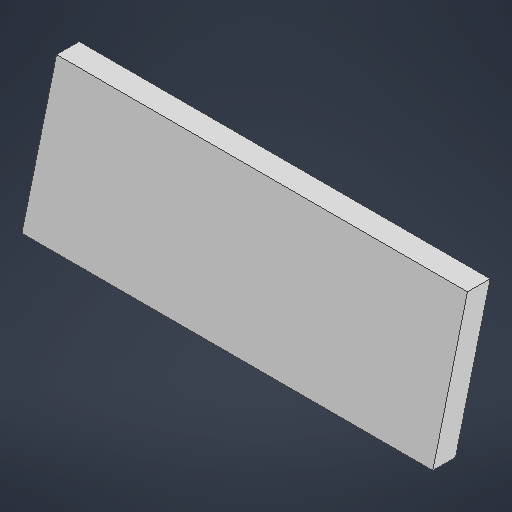
# Autodesk Inventor part: для ведра
Saved by Autodesk Inventor 2025 (Build 290162000, 162)
## iProperties
Created: 2025-03-17
Part Number: для ведра
Material: Типовые
Document SubType Name: Modeling
Designer: Phantom
Density: 1 g/cm^3
Appearance: По умолчанию
Author: Phantom
Autodesk Inventor part; units mm, degrees
ref_plane "YZ Plane" through (0, 0, 0) normal (1, 0, 0) x (0, 1, 0)
ref_plane "XZ Plane" through (0, 0, 0) normal (0, 1, 0) x (-1, 0, 0)
ref_plane "XY Plane" through (0, 0, 0) normal (0, 0, 1) x (1, 0, 0)
sketch "Эскиз1" plane through (0, 0, 0) normal (0, 0, 1) x (1, 0, 0)
  line L0 (0, 0) -> (58, 0)
  line L1 (58, 0) -> (58, 22)
  line L2 (58, 22) -> (0, 22)
  line L3 (0, 22) -> (0, 0)
  dimension "d8" = 58
  constraints: 8 end point, 2 parallel, 1 horizontal, 1 perpendicular
  measures "d8" distance of L0.start L0.end
extrude "Выдавливание1" add sketch "Эскиз1" along normal blind 3.2
sketch "Эскиз2" plane through (0, 0, 0) normal (-1, 0, 0) x (0, 0, 1)
  line L0 (-8.3013, 45.5697) -> (3.4651, -1.0505)
  line L1 (45.6651, 0) -> (-10.7349, 0)
  line L2 (3.4651, 39.7252) -> (31.4651, 39.7252)
  line L3 (31.4651, 39.7252) -> (31.4651, 9.6303)
  line L4 (31.4651, 9.6303) -> (3.4651, 9.6303)
  line L5 (3.4651, 9.6303) -> (3.4651, 39.7252)
  line L6 (-10.7349, 50.4245) -> (-10.7349, 0)
  line L7 (45.6651, 0) -> (-10.7349, 0)
  line L8 (45.6651, 50.4245) -> (45.6651, 0)
  line L9 (45.6651, 50.4245) -> (-10.7349, 50.4245)
  line L10 (3.2, 0) -> (3.2, 22) projected
  line L11 (0, 22) -> (0, 0) projected
  line L12 (0, 0) -> (3.2, 0) projected
  line L13 (3.2, 22) -> (3.2, 0) projected
  line L14 (0, 22) -> (3.2, 22) projected
  point P0 (17.4651, -2.237)
  point P1 (3.2, 0)
  point P2 (0, 12.6789)
  point P3 (3.2, 0)
  constraints: 20 end point, 2 point on line
extrude "Выдавливание2" cut sketch "Эскиз2" against normal through all contours L11 L14 L10 L0
sketch "Эскиз3" plane through (0, 0, 0) normal (-1, 0, 0) x (0, 0, 1)
  line L0 (0, 12.6789) -> (0, 0) projected
  line L1 (3.2, 0) -> (0, 12.6789) projected
  line L2 (0, 12.6789) -> (0, 0) projected
  line L3 (0, 0) -> (3.2, 0) projected
  line L4 (3.2, 0) -> (-1.6943, 19.3919)
  line L5 (-1.6943, 19.3919) -> (-4.8943, 19.3919)
  line L6 (-4.8943, 19.3919) -> (0, 0)
  dimension "d4" = 20
  dimension "d5" = 3.2
  constraints: 6 end point, 1 horizontal
  measures "d4" distance of L1.start L4.end
  measures "d5" distance of L4.end L5.end
extrude "Выдавливание3" add sketch "Эскиз3" against normal blind 58 contours L0 L6 L5 L4
